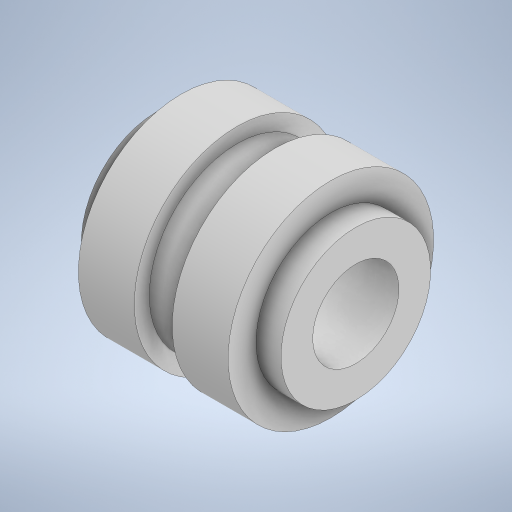
# Autodesk Inventor part: Pieza2-Tarea2
Saved by Autodesk Inventor 2024 (Build 280153000, 153)
## iProperties
Created: 2024-02-22
Part Number: Pieza2-Tarea2
Material: Genérico
Document SubType Name: Modeling
Designer: Diegolap
Density: 1 g/cm^3
Appearance: Valor por defecto
Author: Diegolap
Autodesk Inventor part; units mm, degrees
ref_plane "YZ Plane" through (0, 0, 0) normal (1, 0, 0) x (0, 1, 0)
ref_plane "XZ Plane" through (0, 0, 0) normal (0, 1, 0) x (-1, 0, 0)
ref_plane "XY Plane" through (0, 0, 0) normal (0, 0, 1) x (1, 0, 0)
sketch "Boceto1" plane through (0, 0, 0) normal (0, 0, 1) x (1, 0, 0)
  line L0 (0.1195, 0.0416) -> (6.4695, 0.0416)
  line L1 (6.4695, 0.0416) -> (6.4695, 19.0916)
  line L2 (6.4695, 19.0916) -> (0.1195, 19.0916)
  line L3 (0.1195, 19.0916) -> (0.1195, 0.0416)
  line L4 (6.4695, 0.0416) -> (20.6935, 0.0416)
  line L5 (20.6935, 0.0416) -> (20.6935, 26.2036)
  line L6 (20.6935, 26.2036) -> (6.4695, 26.2036)
  line L7 (6.4695, 26.2036) -> (6.4695, 0.0416)
  line L8 (20.6935, 0.0416) -> (30.3455, 0.0416)
  line L9 (30.3455, 0.0416) -> (30.3455, 22.3936)
  line L10 (30.3455, 22.3936) -> (20.6935, 22.3936)
  line L11 (20.6935, 22.3936) -> (20.6935, 0.0416)
  line L12 (30.3455, 0.0416) -> (44.5695, 0.0416)
  line L13 (44.5695, 0.0416) -> (44.5695, 26.2036)
  line L14 (44.5695, 26.2036) -> (30.3455, 26.2036)
  line L15 (30.3455, 26.2036) -> (30.3455, 0.0416)
  line L16 (44.5695, 0.0416) -> (50.9195, 0.0416)
  line L17 (50.9195, 0.0416) -> (50.9195, 19.0916)
  line L18 (50.9195, 19.0916) -> (44.5695, 19.0916)
  line L19 (44.5695, 19.0916) -> (44.5695, 0.0416)
  line L20 (0.1195, 0.0416) -> (50.9195, 0.0416)
  dimension "d2" = 19.05
  dimension "d3" = 26.162
  dimension "d4" = 9.652
  dimension "d5" = 50.8
  dimension "d6" = 14.224
  dimension "d7" = 6.35
  dimension "d8" = 3.81
  constraints: 42 end point, 10 parallel, 6 horizontal, 5 perpendicular, 2 point on line, 1 collinear
  measures "d2" distance of L2.end L0.start
  measures "d3" distance of L6.end L0.end
  measures "d4" distance of L9.end L10.end
  measures "d5" distance of L2.end L17.end
  measures "d6" distance of L0.end L4.end
  measures "d7" distance of L0.start L0.end
  measures "d8" distance between parallel lines of L14 L10
revolve "Revolución1" add sketch "Boceto1" angle 360 about axis through (0.1195, 0.0416, 0) along (1, 0, 0)
sketch "Boceto2" plane through (0.1195, 0.0416, 0) normal (-1, 0, 0) x (0, 0, 1)
  circle A0 centre (0, -0.0416) radius 10.9883
  constraints: 1 centre point, 1 coincident
extrude "Extrusión1" cut sketch "Boceto2" against normal blind 50.8
equation "\"d2\" = 0.5 * DistC"
equation "\"d3\" = 0.5 * DistA"
equation "\"d4\" = DistE"
equation "\"d5\" = DistB"
equation "\"d6\" = DistX"
equation "\"d7\" = DistD - DistX"
equation "\"d10\" = DistB"
equation "\"DistA\" = 52.324"
equation "\"DistB\" = 50.8"
equation "\"DistC\" = 38.1"
equation "\"DistD\" = 20.574"
equation "\"DistE\" = 9.652"
equation "\"DistX\" = 14.224"
